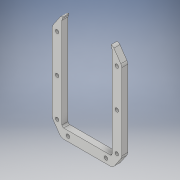
# Autodesk Inventor part: spacer
Saved by Autodesk Inventor 2019 (Build 230136000, 136)
## iProperties
Created: 2019-07-16
Part Number: spacer
Material: Generic
Document SubType Name: Modeling
Designer: Ironic
Density: 1 g/cm^3
Appearance: Default
Author: Ironic
Autodesk Inventor part; units mm, degrees
ref_plane "YZ Plane" through (0, 0, 0) normal (1, 0, 0) x (0, 1, 0)
ref_plane "XZ Plane" through (0, 0, 0) normal (0, 1, 0) x (-1, 0, 0)
ref_plane "XY Plane" through (0, 0, 0) normal (0, 0, 1) x (1, 0, 0)
sketch "Sketch1" plane through (0, 0, 0) normal (0, 0, 1) x (1, 0, 0)
  line L0 (-14.5, 53.5) -> (-14.5, 1)
  line L1 (-20.1, 2.8234) -> (-20.1, 47.0766)
  arc A0 (-20.1, 2.8234) -> (-19.5808, 1.1364) centre (-17.1, 2.8234) ccw
  line L2 (-15.8929, -4.2869) -> (-19.5808, 1.1364)
  arc A1 (-15.8929, -4.2869) -> (-13.4121, -5.6) centre (-13.4121, -2.6) ccw
  line L3 (13.4121, -5.6) -> (-13.4121, -5.6)
  arc A2 (13.4121, -5.6) -> (15.8929, -4.2869) centre (13.4121, -2.6) ccw
  line L4 (19.5808, 1.1364) -> (15.8929, -4.2869)
  line L5 (-13.5, 0) -> (13.5, 0)
  line L6 (14.5, 1) -> (14.5, 53.5)
  arc A3 (13.5, 0) -> (14.5, 1) centre (13.5, 1) ccw
  arc A4 (19.5808, 1.1364) -> (20.1, 2.8234) centre (17.1, 2.8234) ccw
  line L7 (20.1, 47.0766) -> (20.1, 2.8234)
  arc A5 (20.1, 47.0766) -> (19.5808, 48.7636) centre (17.1, 47.0766) ccw
  line L8 (15.5953, 54.6246) -> (19.5808, 48.7636)
  arc A6 (-19.5808, 48.7636) -> (-20.1, 47.0766) centre (-17.1, 47.0766) ccw
  line L9 (-19.5808, 48.7636) -> (-15.5953, 54.6246)
  arc A7 (-13.9414, 55.5) -> (-15.5953, 54.6246) centre (-13.9414, 53.5) ccw
  line L10 (-13.9414, 55.5) -> (-13.9414, 55)
  arc A8 (-13.8229, 55) -> (-14.5, 53.5) centre (-12.5, 53.5) ccw
  arc A9 (15.5953, 54.6246) -> (13.9414, 55.5) centre (13.9414, 53.5) ccw
  line L11 (13.9414, 55.5) -> (13.9414, 55)
  arc A10 (14.5, 53.5) -> (13.8229, 55) centre (12.5, 53.5) ccw
  line L12 (-13.9414, 55) -> (-13.9414, 54.8865)
  arc A11 (-12.5, 55.5) -> (-14.5, 53.5) centre (-12.5, 53.5) ccw
  line L13 (13.9414, 55) -> (13.9414, 54.8865)
  circle A12 centre (17.3, 46.5) radius 1.025
  circle A13 centre (-17.3, 46.5) radius 1.025
  circle A14 centre (-17.3, 24.5) radius 1.025
  circle A15 centre (-17.3, 2.5) radius 1.025
  circle A16 centre (-11, -2.8) radius 1.025
  circle A17 centre (11, -2.8) radius 1.025
  circle A18 centre (17.3, 2.5) radius 1.025
  circle A19 centre (17.3, 24.5) radius 1.025
  arc A20 (-14.5, 1) -> (-13.5, 0) centre (-13.5, 1) ccw
  line L14 (20.1, 47.0766) -> (21.1, 47.0766)
  line L15 (21.1, 47.0766) -> (21.1, 45.0766)
  line L16 (21.1, 45.0766) -> (20.1, 45.0766)
  line L17 (20.1, 45.0766) -> (20.1, 47.0766)
  line L18 (21.1, 45.0766) -> (23.1, 45.0766)
  line L19 (23.1, 45.0766) -> (23.1, 47.0766)
  line L20 (23.1, 47.0766) -> (21.1, 47.0766)
  line L21 (21.1, 47.0766) -> (21.1, 45.0766)
  line L22 (20.1, 2.8234) -> (21.1, 2.8234)
  line L23 (21.1, 2.8234) -> (21.1, 4.8234)
  line L24 (21.1, 4.8234) -> (20.1, 4.8234)
  line L25 (20.1, 4.8234) -> (20.1, 2.8234)
  line L26 (21.1, 4.8234) -> (23.1, 4.8234)
  line L27 (23.1, 4.8234) -> (23.1, 2.8234)
  line L28 (23.1, 2.8234) -> (21.1, 2.8234)
  line L29 (21.1, 2.8234) -> (21.1, 4.8234)
  point P0 (0, 42.5)
  point P1 (0, 0)
  dimension "d2" = 1
  dimension "d3" = 2
  dimension "d4" = 2
  dimension "d5" = 1
  dimension "d6" = 2
  constraints: 60 end point, 28 point on circle, 21 centre point, 8 parallel, 4 horizontal, 4 perpendicular, 2 vertical, 1 midpoint, 1 point on line
  measures "d2" distance of L15.end L16.end
  measures "d3" distance of L14.end L15.end
  measures "d4" distance of L20.end L19.end
  measures "d5" distance of L24.end L23.end
  measures "d6" distance of L23.end L22.end
extrude "Extrusion1" add sketch "Sketch1" along normal blind 3.5 contours L0 A20 L5 A3 L6 A10 L13 L11 A9 L8 A5 L7 A4 L4 A2 L3 A1 L2 A0 L1 A6 L9 A7 L10 L12 A8
body "Solid1"
